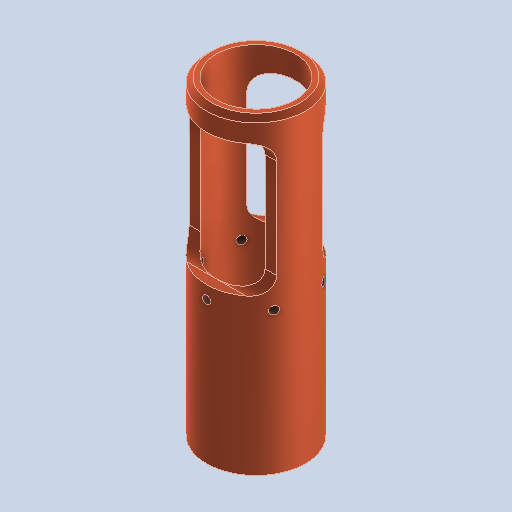
# Autodesk Inventor part: 32
Saved by Autodesk Inventor 2025.1 (Build 291241000, 241)
## iProperties
Created: 2024-09-17
Part Number: 32
Material: Copper
Document SubType Name: Modeling
Designer: ffogue
Density: 8.94 g/cm^3
Appearance: Copper - Satin
Author: ffogue
Autodesk Inventor part; units mm, degrees
ref_plane "XY Plane" through (0, 0, 0) normal (0, 0, 1) x (1, 0, 0)
sketch "Sketch1" plane through (0, 0, 0) normal (0, 0, 1) x (1, 0, 0)
  circle A0 centre (0, 0) radius 15
  circle A1 centre (0, 0) radius 12
  dimension "d0" = 30
  dimension "d1" = 24
  constraints: 2 centre point, 2 coincident
  measures "d0" diameter of A0
  measures "d1" diameter of A1
extrude "Extrusion1" add sketch "Sketch1" against normal blind 94
ref_plane "Work Plane1" through (15, 0, 0) normal (1, 0, 0) x (0, 1, 0)
sketch "Sketch2" plane through (15, 0, 0) normal (1, 0, 0) x (0, 1, 0)
  line L0 (15, 0) -> (15, -94) projected
  line L1 (15, 0) -> (-15, 0) projected
  line L2 (-15, 0) -> (-15, -94) projected
  line L3 (15, -7) -> (7, -7)
  line L4 (7, -7) -> (7, -47)
  line L5 (7, -47) -> (15, -47)
  line L6 (15, -47) -> (15, -7)
  point P0 (0, 0)
  point P1 (11, -7)
  point P2 (0, 0)
  point P3 (15, -27)
  dimension "d5" = 40
  dimension "d6" = 7
  dimension "d8" = 8
  constraints: 8 end point, 3 midpoint, 2 parallel, 1 horizontal, 1 perpendicular, 1 point on line
  measures "d5" distance of L5.end L3.start
  measures "d6" distance between parallel lines of L1 L3
  measures "d8" distance of L3.start L3.end
extrude "Extrusion2" cut sketch "Sketch2" against normal blind 30
mirror "Mirror1" about plane through (0, 0, 0) normal (0, 1, 0) of "Extrusion2"
chamfer "Chamfer1" distance 1.5 angle 45 1 edges at (-15, 0, 0)
fillet "Fillet1" radius 5 8 edges at (-11.5066, 7, -7) (11.5066, 7, -7) (11.5066, -7, -7) (-11.5066, -7, -7) (11.5066, -7, -47) (-11.5066, -7, -47) (-11.5066, 7, -47) (11.5066, 7, -47)
ref_plane "Work Plane2" through (0, 15, 0) normal (0, 1, 0) x (-1, 0, 0)
sketch "Sketch3" plane through (0, 15, 0) normal (0, 1, 0) x (-1, 0, 0)
  line L0 (12, -94) -> (-12, -94) projected
  point P0 (0, 0)
  point P1 (0, -91)
  point P2 (0, -57)
  point P3 (0, -51)
  point P4 (0, -94)
  dimension "d16" = 3
  dimension "d17" = 34
  dimension "d18" = 43
  constraints: 3 vertical alignment, 1 midpoint
  measures "d16" distance from line of L0 point (0, -91)
  measures "d17" distance of point (0, -57) point (0, -91)
  measures "d18" distance from line of L0 point (0, -51)
hole "Hole1" at (0, 15, -91) at (0, 15, -57) direction (0, -1, 0) diameter 4.5 depth 4
hole "Hole2" at (0, 15, -51) direction (0, -1, 0) diameter 2.459 depth 8.8 thread size "M3x0.5" class "6H" standard "ISO Metric profile"
pattern_circular "Circular Pattern1" count 6 over 360 about axis through (0, 0, 0) along (0, 0, -1) of "Hole2"
body "Solid1"
